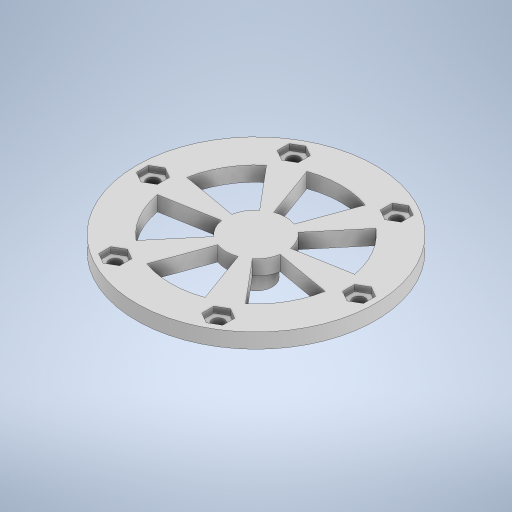
# Autodesk Inventor part: Reaction_wheel
Saved by Autodesk Inventor 2023 (Build 270158000, 158)
## iProperties
Created: 2022-12-10
Part Number: Reaction_wheel
Material: Generic
Document SubType Name: Modeling
Designer: Krzysztof
Density: 1 g/cm^3
Appearance: Default
Author: Krzysztof
Autodesk Inventor part; units mm, degrees
ref_plane "YZ Plane" through (0, 0, 0) normal (1, 0, 0) x (0, 1, 0)
ref_plane "XZ Plane" through (0, 0, 0) normal (0, 1, 0) x (-1, 0, 0)
ref_plane "XY Plane" through (0, 0, 0) normal (0, 0, 1) x (1, 0, 0)
sketch "Sketch1" plane through (0, 0, 0) normal (0, 1, 0) x (-1, 0, 0)
  circle A0 centre (0, 0) radius 80
  line L0 (19.6962, 3.473) -> (56.134, 9.8979)
  line L1 (19.6962, -3.473) -> (56.134, -9.8979)
  line L2 (0, 0) -> (115.9423, 0) construction
  line L3 (0, 0) -> (87.3255, -15.3978) construction
  line L4 (6.8404, 18.7939) -> (19.4951, 53.5625)
  line L5 (12.8558, 15.3209) -> (36.6389, 43.6645)
  line L6 (-12.8558, 15.3209) -> (-36.6389, 43.6645)
  line L7 (-6.8404, 18.7939) -> (-19.4951, 53.5625)
  line L8 (-19.6962, -3.473) -> (-56.134, -9.8979)
  line L9 (-19.6962, 3.473) -> (-56.134, 9.8979)
  line L10 (-6.8404, -18.7939) -> (-19.4951, -53.5625)
  line L11 (-12.8558, -15.3209) -> (-36.6389, -43.6645)
  line L12 (12.8558, -15.3209) -> (36.6389, -43.6645)
  line L13 (6.8404, -18.7939) -> (19.4951, -53.5625)
  arc A1 (56.134, 9.8979) -> (36.6389, 43.6645) centre (0, 0) ccw
  arc A2 (36.6389, -43.6645) -> (56.134, -9.8979) centre (0, 0) ccw
  arc A3 (-19.4951, -53.5625) -> (19.4951, -53.5625) centre (0, 0) ccw
  arc A4 (-56.134, -9.8979) -> (-36.6389, -43.6645) centre (0, 0) ccw
  arc A5 (19.4951, 53.5625) -> (-19.4951, 53.5625) centre (0, 0) ccw
  arc A6 (-36.6389, 43.6645) -> (-56.134, 9.8979) centre (0, 0) ccw
  circle A7 centre (0, 0) radius 57 construction
  circle A8 centre (0, 0) radius 20 construction
  arc A9 (12.8558, -15.3209) -> (19.6962, -3.473) centre (0, 0) ccw
  arc A10 (-6.8404, -18.7939) -> (6.8404, -18.7939) centre (0, 0) ccw
  arc A11 (-19.6962, -3.473) -> (-12.8558, -15.3209) centre (0, 0) ccw
  arc A12 (-12.8558, 15.3209) -> (-19.6962, 3.473) centre (0, 0) ccw
  arc A13 (19.6962, 3.473) -> (12.8558, 15.3209) centre (0, 0) ccw
  arc A14 (6.8404, 18.7939) -> (-6.8404, 18.7939) centre (0, 0) ccw
  dimension "d12" = 40
  dimension "d13" = 114
  dimension "d0" = 160
  dimension "d3" = 20
  dimension "d4" = 10
  dimension "d10" = 360
  constraints: 28 end point, 24 point on circle, 13 centre point, 5 coincident, 1 horizontal, 1 point on line, 44 other
  measures "d0" diameter of A0
  measures "d3" angle of L1 L0
  measures "d4" angle of L2 L3
extrude "Extrusion1" add sketch "Sketch1" against normal blind 10
sketch "Sketch2" plane through (0, 0, 0) normal (0, 1, 0) x (1, 0, 0)
  circle A0 centre (-69, 0) radius 4
  line L0 (0, 0) -> (-95.2262, 0) construction
  line L1 (-69, 8.0829) -> (-62, 4.0415)
  line L2 (-62, 4.0415) -> (-62, -4.0415)
  line L3 (-62, -4.0415) -> (-69, -8.0829)
  line L4 (-69, -8.0829) -> (-76, -4.0415)
  line L5 (-76, -4.0415) -> (-76, 4.0415)
  line L6 (-76, 4.0415) -> (-69, 8.0829)
  line L7 (0, 0) -> (0, 100.6491) construction
  circle A1 centre (-34.5, -59.7558) radius 4
  line L8 (-41.5, -55.7143) -> (-34.5, -51.6728)
  line L9 (-34.5, -51.6728) -> (-27.5, -55.7143)
  line L10 (-27.5, -55.7143) -> (-27.5, -63.7972)
  line L11 (-27.5, -63.7972) -> (-34.5, -67.8387)
  line L12 (-34.5, -67.8387) -> (-41.5, -63.7972)
  line L13 (-41.5, -63.7972) -> (-41.5, -55.7143)
  circle A2 centre (34.5, -59.7558) radius 4
  line L14 (27.5, -63.7972) -> (27.5, -55.7143)
  line L15 (27.5, -55.7143) -> (34.5, -51.6728)
  line L16 (34.5, -51.6728) -> (41.5, -55.7143)
  line L17 (41.5, -55.7143) -> (41.5, -63.7972)
  line L18 (41.5, -63.7972) -> (34.5, -67.8387)
  line L19 (34.5, -67.8387) -> (27.5, -63.7972)
  circle A3 centre (69, 0) radius 4
  line L20 (69, -8.0829) -> (62, -4.0415)
  line L21 (62, -4.0415) -> (62, 4.0415)
  line L22 (62, 4.0415) -> (69, 8.0829)
  line L23 (69, 8.0829) -> (76, 4.0415)
  line L24 (76, 4.0415) -> (76, -4.0415)
  line L25 (76, -4.0415) -> (69, -8.0829)
  circle A4 centre (34.5, 59.7558) radius 4
  line L26 (41.5, 55.7143) -> (34.5, 51.6728)
  line L27 (34.5, 51.6728) -> (27.5, 55.7143)
  line L28 (27.5, 55.7143) -> (27.5, 63.7972)
  line L29 (27.5, 63.7972) -> (34.5, 67.8387)
  line L30 (34.5, 67.8387) -> (41.5, 63.7972)
  line L31 (41.5, 63.7972) -> (41.5, 55.7143)
  circle A5 centre (-34.5, 59.7558) radius 4
  line L32 (-27.5, 63.7972) -> (-27.5, 55.7143)
  line L33 (-27.5, 55.7143) -> (-34.5, 51.6728)
  line L34 (-34.5, 51.6728) -> (-41.5, 55.7143)
  line L35 (-41.5, 55.7143) -> (-41.5, 63.7972)
  line L36 (-41.5, 63.7972) -> (-34.5, 67.8387)
  line L37 (-34.5, 67.8387) -> (-27.5, 63.7972)
  point P0 (-69, 0)
  point P1 (-34.5, -59.7558)
  point P2 (69, 0)
  point P3 (34.5, 59.7558)
  dimension "d16" = 8
  dimension "d17" = 69
  dimension "d18" = 14
  dimension "d21" = 360
  constraints: 76 end point, 6 centre point, 6 coincident, 1 horizontal, 1 parallel, 1 point on line, 1 vertical, 104 other
  measures "d16" diameter of A0
  measures "d17" distance of L0.start A0.centre
  measures "d18" distance between parallel lines of L3 L6
extrude "Extrusion2" cut sketch "Sketch2" against normal blind 4 contours A0 | L1 L2 L3 L4 L5 L6 | A1 | L8 L9 L10 L11 L12 L13 | A2 | L14 L15 L16 L17 L18 L19 | A3 | L20 L21 L22 L23 L24 L25 | A4 | L26 L27 L28 L29 L30 L31 | A5 | L32 L33 L34 L35 L36 L37
extrude "Extrusion3" cut sketch "Sketch2" against normal through all contours A0 | A1 | A2 | A3 | A4 | A5
sketch "Sketch3" plane through (0, -10, 0) normal (0, -1, 0) x (1, 0, 0)
  circle A0 centre (0, 0) radius 11
  dimension "d27" = 22
  constraints: 1 centre point, 1 coincident
  measures "d27" diameter of A0
extrude "Extrusion4" add sketch "Sketch3" along normal blind 15
sketch "Sketch4" plane through (0, -25, 0) normal (0, -1, 0) x (1, 0, 0)
  arc A0 (-1.5, 2) -> (1.5, 2) centre (0, 0) ccw
  line L0 (-1.5, 2) -> (1.5, 2)
  dimension "d30" = 5
  dimension "d31" = 2
  constraints: 2 end point, 2 point on circle, 1 centre point, 1 coincident, 1 horizontal
  measures "d30" diameter of A0
  measures "d31" distance from line of L0 A0.centre
extrude "Extrusion5" cut sketch "Sketch4" against normal blind 20
body "Solid1"
